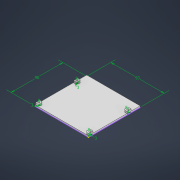
# Autodesk Inventor part: caseBack
Saved by Autodesk Inventor 2021 (Build 250183000, 183)
## iProperties
Created: 2021-08-22
Part Number: caseBack
Material: Generic
Document SubType Name: Modeling
Designer: ryanp
Density: 1 g/cm^3
Appearance: Default
Author: ryanp
Autodesk Inventor part; units mm, degrees
ref_plane "YZ Plane" through (0, 0, 0) normal (1, 0, 0) x (0, 1, 0)
ref_plane "XZ Plane" through (0, 0, 0) normal (0, 1, 0) x (-1, 0, 0)
ref_plane "XY Plane" through (0, 0, 0) normal (0, 0, 1) x (1, 0, 0)
sketch "Sketch1" plane through (0, 0, 0) normal (0, 1, 0) x (-1, 0, 0)
  line L0 (0, 0) -> (93, 0)
  line L1 (93, 0) -> (93, -90)
  line L2 (93, -90) -> (0, -90)
  line L3 (0, -90) -> (0, 0)
  circle A0 centre (90.8, -4.5) radius 1.5
  circle A1 centre (90.8, -70.8) radius 1.5
  circle A2 centre (2.2, -4.5) radius 1.5
  circle A3 centre (2.2, -70.8) radius 1.5
  arc A4 (0, -74.1407) -> (0, -67.4593) centre (2.2, -70.8) ccw
  arc A5 (0, -7.8407) -> (0, -1.1593) centre (2.2, -4.5) ccw
  arc A6 (93, -67.4593) -> (93, -74.1407) centre (90.8, -70.8) ccw
  arc A7 (93, -1.1593) -> (93, -7.8407) centre (90.8, -4.5) ccw
  dimension "d0" = 93
  dimension "d1" = 90
  dimension "d13" = 3
  dimension "d14" = 3
  dimension "d15" = 3
  dimension "d39" = 8
  dimension "d40" = 8
  dimension "d41" = 8
  dimension "d42" = 8
  constraints: 8 centre point, 8 coincident, 8 end point, 8 point on circle, 8 point on line, 2 parallel, 1 horizontal, 1 perpendicular
  measures "d0" distance of L1.end L2.end
  measures "d1" distance of L1.start L1.end
  measures "d13" diameter of A0
  measures "d14" diameter of A1
  measures "d15" diameter of A2
  measures "d39" diameter of A4
  measures "d40" diameter of A5
  measures "d41" diameter of A6
  measures "d42" diameter of A7
extrude "Extrusion6" add sketch "Sketch1" along normal blind 2 contours L0 L1 A7 A6 L2 L3 A4 A5
extrude "Extrusion7" add sketch "Sketch1" along normal blind 5 contours A5 L3 | L1 A7 | A4 L3 | L1 A6
sketch "Sketch4" plane through (0, 0, 0) normal (0, -1, 0) x (1, 0, 0)
  circle A0 centre (-2.2, -4.5) radius 1.5 projected
  circle A1 centre (-2.2, -4.5) radius 3.125
  circle A2 centre (-2.2, -70.8046) radius 3.125
  circle A3 centre (-90.8, -4.5) radius 1.5 projected
  circle A4 centre (-90.8, -4.5) radius 3.125
  circle A5 centre (-90.8, -70.8) radius 1.5 projected
  circle A6 centre (-90.8, -70.8) radius 3.125
  point P0 (0, 0)
  dimension "d47" = 6.25
  dimension "d48" = 6.25
  dimension "d49" = 6.25
  dimension "d50" = 6.25
  constraints: 4 centre point, 3 coincident
  measures "d47" diameter of A1
  measures "d48" diameter of A2
  measures "d49" diameter of A4
  measures "d50" diameter of A6
extrude "Extrusion8" cut sketch "Sketch4" against normal blind 2 contours A0 | A1 | A2 | A4 | A5 | A6
body "Solid3"
